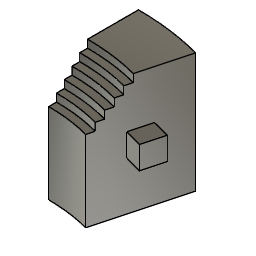
HCDE_Final_Outside_2 v4 (Autodesk Fusion 360 design; units mm, degrees)
Autodesk Fusion 360 part; units mm, degrees
sketch "Sketch1" plane through (0, 0, 0) normal (0, 0, 1) x (1, 0, 0)
  circle A0 centre (0, 0) radius 175
  circle A1 centre (0, 0) radius 212.5
  circle A2 centre (0, 0) radius 137.5
  line L0 (0, 0) -> (54.999, 205.2592)
  line L1 (0, 0) -> (212.5, 0) construction
  line L2 (0, 0) -> (0, 212.5)
  dimension "d1" = 350
  dimension "d2" = 425
  dimension "d3" = 275
  dimension "d4" = 75
  constraint coincident A0.centre A1.centre
  constraint concentric A0 A2
  constraint horizontal L1
  constraint coincident A1 L0.end
  constraint coincident A1 L2.end
  constraint perpendicular L1 L2
  measures "d1" diameter of A0
  measures "d2" diameter of A1
  measures "d3" diameter of A2
  measures "d4" angle of L0 L1
extrude "Extrude13" add sketch "Sketch1" against normal blind 100 contours A0 A2 L0 L2 | A0 A1 L0 L2 picked at (37.0898, 158.0644) picked at (11.2576, 199.5085)
sketch "Sketch12" plane through (0, 0, 0) normal (0, 0, 1) x (-1, 0, 0)
  arc A0 (-54.999, -205.2592) -> (0, -212.5) centre (0, 0) ccw
  line L0 (0, -212.5) -> (0, -137.5)
  arc A1 (-35.5876, -132.8148) -> (0, -137.5) centre (0, 0) ccw
  line L1 (-35.5876, -132.8148) -> (-54.999, -205.2592)
  arc A2 (-43.9992, -164.2074) -> (0, -170) centre (0, 0) ccw
  arc A3 (-42.3169, -157.9289) -> (0, -163.5) centre (0, 0) ccw
  arc A4 (-40.6346, -151.6504) -> (0, -157) centre (0, 0) ccw
  arc A5 (-38.9523, -145.3718) -> (0, -150.5) centre (0, 0) ccw
  arc A6 (-37.2699, -139.0933) -> (0, -144) centre (0, 0) ccw
  dimension "d62" = 170
  dimension "d63" = 163.5
  dimension "d64" = 157
  dimension "d65" = 150.5
  dimension "d66" = 144
  constraint coincident L1 A2.start
  constraint coincident L0 A2.end
  constraint coincident A0.centre A1.centre
  constraint coincident L1 A3.start
  constraint coincident L0 A3.end
  constraint coincident L1 A4.start
  constraint coincident L1 A5.start
  constraint coincident L0 A5.end
  constraint coincident L1 A6.start
  constraint coincident L0 A6.end
  measures "d62" radius of A2
  measures "d63" radius of A3
  measures "d64" radius of A4
  measures "d65" radius of A5
  measures "d66" radius of A6
extrude "Extrude14" cut sketch "Sketch12" against normal blind 6.5 contours L0 L1 A2 A3
extrude "Extrude15" cut sketch "Sketch12" against normal blind 13 contours L0 L1 A3 A4
extrude "Extrude16" cut sketch "Sketch12" against normal blind 19.5 contours L0 L1 A4 A5
extrude "Extrude17" cut sketch "Sketch12" against normal blind 26 contours L0 L1 A5 A6
extrude "Extrude18" cut sketch "Sketch12" against normal blind 32.5 contours L0 A1 L1 A6
sketch "Sketch15" plane through (0, 0, 0) normal (-1, 0, 0) x (0, -1, 0)
  line L0 (-137.5, -32.5) -> (-144, -32.5)
  line L1 (-144, -32.5) -> (-144, -26)
  line L2 (-144, -26) -> (-150.5, -26)
  line L3 (-150.5, -26) -> (-150.5, -19.5)
  line L4 (-150.5, -19.5) -> (-157, -19.5)
  line L5 (-157, -19.5) -> (-157, -13)
  line L6 (-157, -13) -> (-163.5, -13)
  line L7 (-163.5, -13) -> (-163.5, -6.5)
  line L8 (-163.5, -6.5) -> (-170, -6.5)
  line L9 (-170, -6.5) -> (-170, 0)
  line L10 (-170, 0) -> (-212.5, 0)
  line L11 (-212.5, 0) -> (-212.5, -100)
  line L12 (-212.5, -100) -> (-137.5, -100)
  line L13 (-137.5, -100) -> (-137.5, -32.5)
  line L14 (-164.5, -39.5) -> (-185.5, -39.5)
  line L15 (-185.5, -39.5) -> (-185.5, -60.5)
  line L16 (-185.5, -60.5) -> (-164.5, -60.5)
  line L17 (-164.5, -60.5) -> (-164.5, -39.5)
  point P0 (-175, -50)
  point P1 (-175, -50)
  dimension "d77" = 50
  dimension "d78" = 37.5
  dimension "d79" = 21
  dimension "d88" = 10.5
  dimension "d89" = 10.5
  dimension "d90" = 10.5
  constraint horizontal L14
  constraint perpendicular L14 L15
  constraint parallel L14 L16
  constraint parallel L15 L17
  constraint coincident P1 P0
  measures "d77" distance of L10 P1
  measures "d78" distance of L11 P1
  measures "d79" distance of L15.end L16.end
  measures "d88" distance of L17 P1
  measures "d89" distance of L14 P1
  measures "d90" distance of L16 P1
extrude "Extrude19" cut sketch "Sketch15" against normal blind 15 contours L14 L15 L16 L17
sketch "Sketch16" plane through (0, 0, 0) normal (0.965926, -0.258819, 0) x (0.258819, 0.965926, 0)
  line L0 (144, -32.5) -> (137.5, -32.5)
  line L1 (137.5, -32.5) -> (137.5, -100)
  line L2 (137.5, -100) -> (212.5, -100)
  line L3 (212.5, -100) -> (212.5, 0)
  line L4 (212.5, 0) -> (170, 0)
  line L5 (170, 0) -> (170, -6.5)
  line L6 (170, -6.5) -> (163.5, -6.5)
  line L7 (163.5, -6.5) -> (163.5, -13)
  line L8 (163.5, -13) -> (157, -13)
  line L9 (157, -13) -> (157, -19.5)
  line L10 (157, -19.5) -> (150.5, -19.5)
  line L11 (150.5, -19.5) -> (150.5, -26)
  line L12 (150.5, -26) -> (144, -26)
  line L13 (144, -26) -> (144, -32.5)
  line L14 (184.5, -40.5) -> (165.5, -40.5)
  line L15 (165.5, -40.5) -> (165.5, -59.5)
  line L16 (165.5, -59.5) -> (184.5, -59.5)
  line L17 (184.5, -59.5) -> (184.5, -40.5)
  point P0 (175, -50)
  point P1 (175, -50)
  dimension "d82" = 50
  dimension "d83" = 37.5
  dimension "d84" = 19
  dimension "d91" = 9.5
  dimension "d92" = 9.5
  dimension "d93" = 9.5
  constraint horizontal L14
  constraint perpendicular L14 L15
  constraint parallel L14 L16
  constraint parallel L15 L17
  constraint coincident P1 P0
  measures "d82" distance of L4 P1
  measures "d83" distance of L3 P1
  measures "d84" distance of L15.end L16.end
  measures "d91" distance of P1 L17
  measures "d92" distance of P1 L14
  measures "d93" distance of L16 P1
extrude "Extrude20" add sketch "Sketch16" along normal blind 15 contours L14 L15 L16 L17
shell "Shell4" thickness 2 removed faces 1 at (42.4956, 182.4486, -100)
sketch "Sketch13" plane through (0, 0, 0) normal (0, 0, 1) x (-1, 0, 0)
sketch "Sketch14" plane through (0, 0, 0) normal (0, 0, 1) x (-1, 0, 0)
extrude "Extrude1" [suppressed]
chamfer "Chamfer1" [suppressed]
ref_plane "WorkPlane2" through (0, 0, 0) normal (0, 0, 1) x (1, 0, 0)
sketch "Sketch2" plane through (0, 0, 0) normal (1, 0, 0) x (0, 1, 0)
  line L0 (137.5, -32.5) -> (137.5, -100)
  line L1 (212.5, 0) -> (170, 0)
  line L2 (165, -40) -> (185, -40)
  line L3 (185, -40) -> (185, -60)
  line L4 (185, -60) -> (165, -60)
  line L5 (165, -60) -> (165, -40)
  point P0 (175, -50)
  point P1 (175, -50)
  dimension "d8" = 37.5
  dimension "d9" = 50
  dimension "d10" = 20
  dimension "d11" = 20
  constraint horizontal L2
  constraint perpendicular L2 L3
  constraint parallel L2 L4
  constraint parallel L3 L5
  constraint coincident P0 P1
  measures "d8" distance of P0 L0
  measures "d9" distance of P0 L1
  measures "d10" distance of L3.end L4.end
  measures "d11" distance of L2.end L3.end
extrude "Extrude2" [suppressed]
ref_plane "WorkPlane1" through (87.5, 151.5544, -50) normal (0.866025, -0.5, 0) x (-0.5, -0.866025, 0)
sketch "Sketch3" plane through (0, 0, 0) normal (0.866025, -0.5, 0) x (-0.5, -0.866025, 0)
  line L0 (-212.5, 0) -> (-212.5, 100)
  line L1 (-212.5, 100) -> (-137.5, 100)
  line L2 (-185, 40) -> (-165, 40)
  line L3 (-165, 40) -> (-165, 60)
  line L4 (-165, 60) -> (-185, 60)
  line L5 (-185, 60) -> (-185, 40)
  point P0 (-175, 50)
  point P1 (-175, 50)
  dimension "d15" = 37.5
  dimension "d16" = 50
  dimension "d17" = 20
  dimension "d18" = 20
  constraint horizontal L2
  constraint perpendicular L2 L3
  constraint parallel L2 L4
  constraint parallel L3 L5
  constraint coincident P0 P1
  measures "d15" distance of P0 L0
  measures "d16" distance of P0 L1
  measures "d17" distance of L3.end L4.end
  measures "d18" distance of L2.end L3.end
extrude "Extrude3" [suppressed]
sketch "Sketch7" plane through (0, 0, 0) normal (0, 0, 1) x (-1, 0, 0)
  arc A0 (-85, -147.2243) -> (-0.1035, -170) centre (0, 0) ccw
  line L0 (-85, -147.2243) -> (-106.25, -184.0304)
  arc A1 (-106.25, -184.0304) -> (-0.1035, -212.5) centre (0, 0) ccw
  line L1 (-0.1035, -212.5) -> (-0.1035, -170)
  arc A2 (-101.625, -176.0197) -> (-0.1047, -203.25) centre (0, 0) ccw
  arc A3 (-89.625, -155.2351) -> (-0.101, -179.25) centre (0, 0) ccw
  line L2 (0, 0) -> (200, 0) construction
  line L3 (0, 0) -> (-85.8972, -184.2071)
  line L4 (0, 0) -> (200, 0) construction
  line L5 (0, 0) -> (200, 0) construction
  line L6 (0, 0) -> (203.25, 0) construction
  line L7 (0, 0) -> (-17.7144, -202.4766)
  line L8 (0, 0) -> (203.25, 0) construction
  point P0 (-49.5488, -184.72)
  point P1 (-49.5488, -184.72)
  dimension "d34" = 203.25
  dimension "d35" = 179.25
  dimension "d37" = 115
  dimension "d38" = 203.25
  dimension "d43" = 95
  constraint coincident L0 A2.start
  constraint coincident A0.centre A1.centre
  constraint coincident L0 A3.start
  constraint horizontal L2
  constraint horizontal L4
  constraint horizontal L5
  constraint horizontal L6
  constraint horizontal L8
  constraint coincident P1 P0
  measures "d34" radius of A2
  measures "d35" radius of A3
  measures "d37" angle of L3 L4
  measures "d38" distance of A0.centre L3.end
  measures "d43" angle of L7 L8
extrude "Extrude7" [suppressed]
ref_plane "WorkPlane4" through (50.7599, 182.4661, -7) normal (0, 0, 1) x (-1, 0, 0)
sketch "Sketch8" plane through (0, 0, -7) normal (0, 0, 1) x (1, 0, 0)
ref_plane "WorkPlane5" through (50.7599, 182.4661, -7) normal (0, 0, 1) x (-1, 0, 0)
sketch "Sketch9" plane through (0, 0, -7) normal (0, 0, 1) x (1, 0, 0)
sketch "Sketch10" plane through (0, 0, -7) normal (0, 0, 1) x (-1, 0, 0)
  line L0 (-75.7543, -162.4557) -> (-85.8972, -184.2071)
  arc A0 (-85.8972, -184.2071) -> (-17.7144, -202.4766) centre (0, 0) ccw
  line L1 (-17.7144, -202.4766) -> (-15.6227, -178.5679)
  arc A1 (-75.7543, -162.4557) -> (-15.6227, -178.5679) centre (0, 0) ccw
  circle A2 centre (-49.5488, -184.72) radius 12
  point P0 (-49.5488, -184.72)
  dimension "d46" = 24
  constraint coincident P0 A2.centre
  measures "d46" diameter of A2
extrude "Extrude8" [suppressed]
sketch "Sketch11" plane through (0, 0, -15) normal (0, 0, 1) x (-1, 0, 0)
  circle A0 centre (-49.5488, -184.72) radius 12
  circle A1 centre (-49.5488, -184.72) radius 7.5
  point P0 (-49.5488, -184.72)
  dimension "d49" = 15
  constraint concentric A0 A1
  measures "d49" diameter of A1
extrude "Extrude9" [suppressed]
shell "Shell3" [suppressed]
extrude "Extrude10" [suppressed]
extrude "Extrude11" [suppressed]
